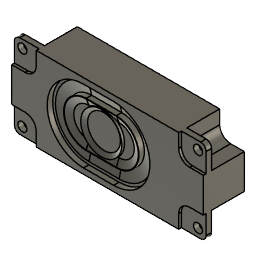
Senso v45 (Autodesk Fusion 360 archive; units mm, degrees)
design "Speaker"
Autodesk Fusion 360 part; units mm, degrees
sketch "Sketch1" plane through (0, 0, 0) normal (0, 1, 0) x (1, 0, 0)
  line L0 (2, 0) -> (68, 0)
  line L1 (70, -2) -> (70, -28.6)
  line L2 (68, -30.6) -> (0, -30.6)
  line L3 (0, -28.6) -> (0, -2)
  circle A0 centre (2.95, -27.65) radius 1.65
  circle A1 centre (2.95, -2.95) radius 1.65
  circle A2 centre (67.05, -27.65) radius 1.65
  circle A3 centre (67.05, -2.95) radius 1.65
  line L4 (2, -30.6) -> (9, -30.6)
  line L5 (9, -30.6) -> (9, -25.6)
  line L6 (5, -21.6) -> (0, -21.6)
  line L7 (0, -21.6) -> (0, -30.6)
  arc A4 (9, -25.6) -> (5, -21.6) centre (5, -25.6) ccw
  line L8 (0, -15.3) -> (70, -15.3) construction
  line L9 (35, -30.6) -> (35, 0) construction
  line L10 (5, -9) -> (0, -9)
  arc A5 (5, -9) -> (9, -5) centre (5, -5) ccw
  line L11 (9, 0) -> (9, -5)
  line L12 (65, -21.6) -> (70, -21.6)
  arc A6 (65, -21.6) -> (61, -25.6) centre (65, -25.6) ccw
  line L13 (61, -30.6) -> (61, -25.6)
  line L14 (65, -9) -> (70, -9)
  arc A7 (61, -5) -> (65, -9) centre (65, -5) ccw
  line L15 (61, 0) -> (61, -5)
  arc A8 (0, -28.6) -> (2, -30.6) centre (2, -28.6) ccw
  arc A9 (2, 0) -> (0, -2) centre (2, -2) ccw
  arc A10 (70, -2) -> (68, 0) centre (68, -2) ccw
  arc A11 (68, -30.6) -> (70, -28.6) centre (68, -28.6) ccw
  line L16 (26.25, -28.55) -> (37.25, -28.55)
  line L17 (37.25, -2.05) -> (26.25, -2.05)
  arc A12 (13, -15.3) -> (26.25, -28.55) centre (26.25, -15.3) ccw
  arc A13 (26.25, -2.05) -> (13, -15.3) centre (26.25, -15.3) ccw
  arc A14 (37.25, -28.55) -> (50.5, -15.3) centre (37.25, -15.3) ccw
  arc A15 (50.5, -15.3) -> (37.25, -2.05) centre (37.25, -15.3) ccw
  arc A16 (18, -15.3) -> (26.25, -23.55) centre (26.25, -15.3) ccw
  line L18 (26.25, -23.55) -> (37.25, -23.55)
  arc A17 (37.25, -23.55) -> (45.5, -15.3) centre (37.25, -15.3) ccw
  arc A18 (45.5, -15.3) -> (37.25, -7.05) centre (37.25, -15.3) ccw
  line L19 (37.25, -7.05) -> (26.25, -7.05)
  arc A19 (26.25, -7.05) -> (18, -15.3) centre (26.25, -15.3) ccw
  arc A20 (14, -15.3) -> (26.25, -27.55) centre (26.25, -15.3) ccw
  line L20 (26.25, -27.55) -> (37.25, -27.55)
  arc A21 (37.25, -27.55) -> (49.5, -15.3) centre (37.25, -15.3) ccw
  arc A22 (49.5, -15.3) -> (37.25, -3.05) centre (37.25, -15.3) ccw
  line L21 (37.25, -3.05) -> (26.25, -3.05)
  arc A23 (26.25, -3.05) -> (14, -15.3) centre (26.25, -15.3) ccw
  line L22 (26.25, -15.3) -> (37.25, -15.3)
  circle A24 centre (31.75, -15.3) radius 7.5
  line L23 (37.25, -7.25) -> (26.25, -7.25)
  arc A25 (26.25, -7.25) -> (18.2, -15.3) centre (26.25, -15.3) ccw
  arc A26 (18.2, -15.3) -> (26.25, -23.35) centre (26.25, -15.3) ccw
  line L24 (26.25, -23.35) -> (37.25, -23.35)
  arc A27 (37.25, -23.35) -> (45.3, -15.3) centre (37.25, -15.3) ccw
  arc A28 (45.3, -15.3) -> (37.25, -7.25) centre (37.25, -15.3) ccw
  circle A29 centre (31.75, -15.3) radius 6
  point P0 (70, 0)
  point P1 (13, -28.55)
  point P2 (50.5, -28.55)
  point P3 (13, -2.05)
  dimension "d1" = 70
  dimension "d2" = 30.6
  dimension "d5" = 3.3
  dimension "d6" = 2.95
  dimension "d7" = 2.95
  dimension "d12" = 3.3
  dimension "d13" = 2.95
  dimension "d14" = 2.95
  dimension "d15" = 3.3
  dimension "d16" = 3.3
  dimension "d17" = 2.95
  dimension "d18" = 2.95
  dimension "d19" = 2.95
  dimension "d20" = 2.95
  dimension "d21" = 9
  dimension "d22" = 9
  dimension "d23" = 4
  dimension "d28" = 2
  dimension "d31" = 37.5
  dimension "d32" = 26.5
  dimension "d34" = 13.25
  dimension "d35" = 13.25
  dimension "d36" = 13.25
  dimension "d37" = 13.25
  dimension "d38" = -5
  dimension "d43" = -1
  dimension "d48" = 15
  dimension "d49" = -0.2
  dimension "d54" = 12
  constraint horizontal L0
  constraint vertical L1
  constraint horizontal L2
  constraint vertical L3
  constraint horizontal L4
  constraint vertical L5
  constraint horizontal L6
  constraint vertical L7
  constraint tangent L6 A4
  constraint tangent L5 A4
  constraint symmetric L4.end L8 L11.start
  constraint symmetric L6.end L8 L10.end
  constraint symmetric L6.start L8 L10.start
  constraint symmetric L5.end L8 A5.end
  constraint symmetric A4 L8 A5
  constraint symmetric L4.end L9 L13.start
  constraint symmetric L6.end L9 L12.end
  constraint symmetric L6.start L9 L12.start
  constraint symmetric L5.end L9 A6.end
  constraint symmetric A4 L9 A6
  constraint symmetric L9 L10.start L14.start
  constraint symmetric L9 L10.end L14.end
  constraint symmetric L9 A5.end A7.start
  constraint symmetric L9 A5 A7
  constraint symmetric L9 L11.start L15.start
  constraint coincident L3 L8.start
  constraint coincident L2.end L4
  constraint tangent L4 A8
  constraint tangent L3 A8
  constraint coincident L0 L9.end
  constraint coincident origin L3
  constraint coincident origin L0
  constraint tangent L3 A9
  constraint tangent L0 A9
  constraint equal A8 A9
  constraint coincident L1 L8.end
  constraint coincident P0 L0
  constraint coincident P0 L1
  constraint tangent L0 A10
  constraint tangent L1 A10
  constraint equal A8 A10
  constraint coincident L2 L9.start
  constraint tangent L1 A11
  constraint tangent L2 A11
  constraint equal A8 A11
  constraint horizontal L16
  constraint horizontal L17
  constraint coincident P1 L16
  constraint tangent L16 A12
  constraint coincident P3 L17
  constraint tangent L17 A13
  constraint coincident A12.start A13.end
  constraint coincident P2 L16
  constraint tangent L16 A14
  constraint tangent L17 A15
  constraint coincident A14.end A15.start
  constraint coincident A12.centre A13.centre
  constraint coincident A14.centre A15.centre
  constraint perpendicular L9 L22
  constraint midpoint L22 A24.centre
  constraint concentric A24 A29
  measures "d1" distance of origin P0
  measures "d2" distance of origin L2.end
  measures "d5" diameter of A0
  measures "d6" distance of L3 A0.centre
  measures "d7" distance of L2 A0.centre
  measures "d12" diameter of A1
  measures "d13" distance of L3 A1.centre
  measures "d14" distance of L0 A1.centre
  measures "d15" diameter of A2
  measures "d16" diameter of A3
  measures "d17" distance of L1 A3.centre
  measures "d18" distance of L0 A3.centre
  measures "d19" distance of L1 A2.centre
  measures "d20" distance of L2 A2.centre
  measures "d21" distance of L2.end L4.end
  measures "d22" distance of L2.end L6.end
  measures "d23" radius of A4
  measures "d28" radius of A8
  measures "d31" distance of P1 P2
  measures "d32" distance of P1 P3
  measures "d34" radius of A12
  measures "d35" radius of A13
  measures "d36" radius of A14
  measures "d37" radius of A15
  measures "d48" diameter of A24
  measures "d54" diameter of A29
extrude "Extrude1" add sketch "Sketch1" along normal blind 15 contours L0 L1 L2 L3 L5 L6 A4 L10 A5 L11 L12 A6 L13 L14 A7 L15 | L16 L17 A12 A13 A14 A15 | A16 L18 A17 A18 L19 A19 | A20 L20 A21 A22 L21 A23 | A24 | L23 A25 A26 L24 A27 A28 | A29
extrude "Extrude2" add sketch "Sketch1" along normal blind 3 contours L0 L3 L10 A5 L11 A9 | L0 L1 L14 A7 L15 A10 | L2 L3 L4 L5 L6 L7 A4 A8 | L1 L2 L12 A6 L13 A11
extrude "Extrude3" cut sketch "Sketch1" along normal blind 1 contours L0 L3 L10 A5 L11 A9 | L0 L1 L14 A7 L15 A10 | L2 L3 L4 L5 L6 L7 A4 A8 | L1 L2 L12 A6 L13 A11
extrude "Extrude4" cut sketch "Sketch1" along normal blind 2 contours L16 L17 A12 A13 A14 A15 | A20 L20 A21 A22 L21 A23
extrude "Extrude5" cut sketch "Sketch1" along normal blind 1 contours A16 L18 A17 A18 L19 A19 | A24 | L23 A25 A26 L24 A27 A28 | A29
extrude "Extrude6" cut sketch "Sketch1" along normal blind 3 contours A20 L20 A21 A22 L21 A23
chamfer "Chamfer1" distance 1 distance2 4 4 edges at (31.75, 3, 27.55) (49.5, 3, 15.3) (31.75, 3, 3.05) (14, 3, 15.3) measured on face at (29.9167, 2.3333, 27.55) measured on face at (45.1241, 2.6667, 24.684) measured on face at (33.5833, 2.3333, 3.05) measured on face at (17.0652, 2.3333, 23.4057)
extrude "Extrude7" cut sketch "Sketch1" along normal blind 2 contours L23 A25 A26 L24 A27 A28
chamfer "Chamfer2" distance 1 distance2 2.5 4 edges at (31.75, 2, 23.35) (45.3, 2, 15.3) (31.75, 2, 7.25) (18.2, 2, 15.3) measured on face at (29.9167, 1.3333, 23.35) measured on face at (38.0515, 1.3333, 7.29) measured on face at (33.5833, 1.3333, 7.25) measured on face at (18.5009, 1.3333, 17.4803)
extrude "Extrude8" cut sketch "Sketch1" along normal blind 2 contours A29
chamfer "Chamfer3" distance 1.5 distance2 1 1 edges at (26.156, 1, 17.4697) measured on face at (38.7221, 1, 14.9274)
equation "d6 = 1.3 mm + ( 3.3 / 2 ) * 1 mm"
equation "d34 = ( 26.5 / 2 ) * 1 mm"
equation "d35 = ( 26.5 / 2 ) * 1 mm"
equation "d36 = ( 26.5 / 2 ) * 1 mm"
equation "d37 = ( 26.5 / 2 ) * 1 mm"
equation "d54 = 15 mm - 3 mm"

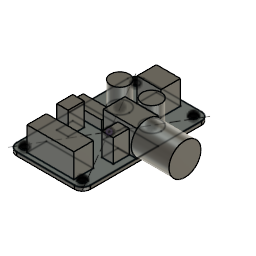
design "Fasizi AudioVerstaerker PAM8406"
Autodesk Fusion 360 part; units mm, degrees
sketch "Sketch1" plane through (0, 0, 0) normal (0, 0, 1) x (1, 0, 0)
  line L0 (12.63, 27.8) -> (-12.63, 27.8)
  line L1 (-16.13, 24.3) -> (-16.13, -24.3)
  line L2 (-12.63, -27.8) -> (12.63, -27.8)
  line L3 (16.13, -24.3) -> (16.13, 24.3)
  line L4 (16.13, 27.8) -> (-16.13, -27.8) construction
  line L5 (-16.13, 27.8) -> (16.13, -27.8) construction
  circle A0 centre (-12.63, 24.3) radius 1.5
  circle A1 centre (12.63, 24.3) radius 1.5
  circle A2 centre (-12.63, -24.3) radius 1.5
  circle A3 centre (12.63, -24.3) radius 1.5
  arc A4 (-12.63, 27.8) -> (-16.13, 24.3) centre (-12.63, 24.3) ccw
  arc A5 (16.13, 24.3) -> (12.63, 27.8) centre (12.63, 24.3) ccw
  arc A6 (12.63, -27.8) -> (16.13, -24.3) centre (12.63, -24.3) ccw
  arc A7 (-16.13, -24.3) -> (-12.63, -27.8) centre (-12.63, -24.3) ccw
  line L6 (-4.63, 25.3) -> (5.87, 25.3)
  line L7 (5.87, 25.3) -> (5.87, 16.8)
  line L8 (5.87, 16.8) -> (-4.63, 16.8)
  line L9 (-4.63, 16.8) -> (-4.63, 25.3)
  circle A8 centre (-6.98, 11.65) radius 4.15
  circle A9 centre (6.98, 11.65) radius 4.15
  line L10 (-16.13, 4.8) -> (-2.13, 4.8)
  line L11 (-2.13, 4.8) -> (-2.13, -1.2)
  line L12 (-2.13, -1.2) -> (-16.13, -1.2)
  line L13 (-16.13, -1.2) -> (-16.13, 4.8)
  line L14 (16.13, 5.3) -> (1.63, 5.3)
  line L15 (1.63, 5.3) -> (1.63, -4.2)
  line L16 (1.63, -4.2) -> (16.13, -4.2)
  line L17 (16.13, -4.2) -> (16.13, 5.3)
  line L18 (-12.13, -3.8) -> (-7.13, -3.8)
  line L19 (-7.13, -3.8) -> (-7.13, -10.8)
  line L20 (-7.13, -10.8) -> (-12.13, -10.8)
  line L21 (-12.13, -10.8) -> (-12.13, -3.8)
  line L22 (8.13, -11.3) -> (13.13, -11.3)
  line L23 (13.13, -11.3) -> (13.13, -4.3)
  line L24 (13.13, -4.3) -> (8.13, -4.3)
  line L25 (8.13, -4.3) -> (8.13, -11.3)
  line L26 (-10.13, -17.3) -> (10.37, -17.3)
  line L27 (10.37, -17.3) -> (10.37, -25.8)
  line L28 (10.37, -25.8) -> (-10.13, -25.8)
  line L29 (-10.13, -25.8) -> (-10.13, -17.3)
  dimension "d1" = 32.26
  dimension "d2" = 55.6
  dimension "d3" = 3
  dimension "d4" = 3.5
  dimension "d5" = 3.5
  dimension "d8" = 25.26
  dimension "d9" = -48.6
  dimension "d10" = 3.5
  dimension "d13" = 10.5
  dimension "d14" = 8.5
  dimension "d15" = 11.5
  dimension "d16" = 2.5
  dimension "d19" = 8.3
  dimension "d20" = 8.3
  dimension "d21" = 9.15
  dimension "d22" = 9.15
  dimension "d23" = 16.15
  dimension "d24" = 16.15
  dimension "d27" = 14
  dimension "d28" = 6
  dimension "d29" = 23
  dimension "d32" = 14.5
  dimension "d33" = 9.5
  dimension "d36" = 5
  dimension "d37" = 7
  dimension "d38" = 4
  dimension "d39" = 17
  dimension "d40" = 22.5
  dimension "d41" = 5
  dimension "d42" = 7
  dimension "d43" = 3
  dimension "d44" = 16.5
  dimension "d47" = 20.5
  dimension "d48" = 8.5
  dimension "d49" = 6
  dimension "d52" = 2
  constraint horizontal L0
  constraint perpendicular L0 L1
  constraint parallel L0 L2
  constraint parallel L1 L3
  constraint coincident L4 origin
  constraint coincident L5 origin
  constraint coincident L5.start L1
  constraint coincident L5.start L0
  constraint tangent L1 A4
  constraint tangent L0 A4
  constraint coincident L4.start L0
  constraint coincident L4.start L3
  constraint tangent L0 A5
  constraint tangent L3 A5
  constraint equal A4 A5
  constraint coincident L5.end L3
  constraint coincident L5.end L2
  constraint tangent L3 A6
  constraint tangent L2 A6
  constraint equal A4 A6
  constraint coincident L4.end L1
  constraint coincident L4.end L2
  constraint tangent L1 A7
  constraint tangent L2 A7
  constraint equal A4 A7
  constraint horizontal L6
  constraint vertical L7
  constraint horizontal L8
  constraint vertical L9
  constraint horizontal L10
  constraint vertical L11
  constraint horizontal L12
  constraint vertical L13
  constraint coincident L1 L10.start
  constraint horizontal L14
  constraint vertical L15
  constraint horizontal L16
  constraint vertical L17
  constraint coincident L3 L14.start
  constraint horizontal L18
  constraint vertical L19
  constraint horizontal L20
  constraint vertical L21
  constraint horizontal L22
  constraint vertical L23
  constraint horizontal L24
  constraint vertical L25
  constraint horizontal L26
  constraint vertical L27
  constraint horizontal L28
  constraint vertical L29
  measures "d1" distance of L4.end L5.end
  measures "d2" distance of L5.start L4.end
  measures "d3" diameter of A0
  measures "d4" distance of L1 A0.centre
  measures "d5" distance of L0 A0.centre
  measures "d10" radius of A4
  measures "d13" distance of L6.start L6.end
  measures "d14" distance of L6.start L8.end
  measures "d15" distance of L1 L9
  measures "d16" distance of L0 L6
  measures "d19" diameter of A8
  measures "d20" diameter of A9
  measures "d21" distance of L1 A8.centre
  measures "d22" distance of L3 A9.centre
  measures "d23" distance of L0 A9.centre
  measures "d24" distance of L0 A8.centre
  measures "d27" distance of L10.start L10.end
  measures "d28" distance of L10.start L12.end
  measures "d29" distance of L0 L10
  measures "d32" distance of L14.start L14.end
  measures "d33" distance of L14.start L16.end
  measures "d36" distance of L18.start L18.end
  measures "d37" distance of L18.start L20.end
  measures "d38" distance of L1 L21
  measures "d39" distance of L2 L20
  measures "d40" distance of L0 L14
  measures "d41" distance of L22.start L22.end
  measures "d42" distance of L22.start L24.end
  measures "d43" distance of L3 L23
  measures "d44" distance of L2 L22
  measures "d47" distance of L26.start L26.end
  measures "d48" distance of L26.start L28.end
  measures "d49" distance of L1 L29
  measures "d52" distance of L2 L28
extrude "Extrude1" add sketch "Sketch1" against normal blind 1.6 contours L0 L1 L2 L3 A4 A5 A6 A7 L10 L11 L12 L14 L15 L16 | L3 L14 L15 L16 L17 | L1 L10 L11 L12 L13 | L6 L7 L8 L9 | A8 | A9 | L18 L19 L20 L21 | L22 L23 L24 L25 | L26 L27 L28 L29 makes body 1
extrude "Extrude2" add sketch "Sketch1" along normal blind 10.5 separate body contours L6 L7 L8 L9 makes body 2
extrude "Extrude3" add sketch "Sketch1" along normal blind 10.5 separate body contours A8 | A9 makes body 3 at (-2.8352, 11.4431, 7) makes body 4 at (11.1248, 11.4431, 7)
extrude "Extrude4" add sketch "Sketch1" along normal blind 4 separate body contours L1 L10 L11 L12 L13 makes body 5
extrude "Extrude5" add sketch "Sketch1" along normal blind 11.5 separate body contours L3 L14 L15 L16 L17 makes body 6
extrude "Extrude6" add sketch "Sketch1" along normal blind 10 separate body contours L18 L19 L20 L21 | L22 L23 L24 L25 makes body 7 at (13.13, -8.9667, 3.3333) makes body 8 at (-7.13, -6.1333, 3.3333)
extrude "Extrude7" add sketch "Sketch1" along normal blind 10.5 separate body contours L26 L27 L28 L29 makes body 9
sketch "Sketch2" plane through (16.13, 0, 0) normal (1, 0, 0) x (0, 1, 0)
  line L0 (-4.2, 0) -> (5.3, 0)
  line L1 (5.3, 0) -> (5.3, 11.5)
  line L2 (5.3, 11.5) -> (-4.2, 11.5)
  line L3 (-4.2, 11.5) -> (-4.2, 0)
  circle A0 centre (0.55, 5.75) radius 7
  dimension "d55" = 14
  measures "d55" diameter of A0
extrude "Extrude8" add sketch "Sketch2" along normal blind 16.5 contours L0 L1 L2 L3 A0 | L0 A0 | L3 A0 | L1 A0 | L2 A0 bodies 1 6
equation "d4 = 2 mm + 1.5 mm"
equation "d5 = 2 mm + 1.5 mm"
equation "d8 = 32.26 mm - ( 3.5 * 2 ) * 1 mm"
equation "d9 = -55.6 mm + ( 3.5 * 2 ) * 1 mm"
equation "d21 = 5 mm + ( 8.3 / 2 ) * 1 mm"
equation "d23 = 12 mm + ( 8.3 / 2 ) * 1 mm"

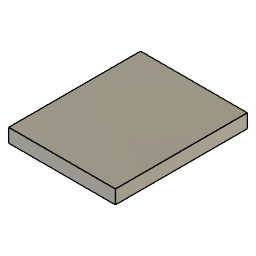
design "LP605060JU Akku"
Autodesk Fusion 360 part; units mm, degrees
sketch "Sketch1" plane through (0, 0, 0) normal (0, 0, 1) x (1, 0, 0)
  line L0 (0, 0) -> (51, 0)
  line L1 (51, 0) -> (51, 63)
  line L2 (51, 63) -> (0, 63)
  line L3 (0, 63) -> (0, 0)
  dimension "d1" = 51
  dimension "d2" = 63
  constraint horizontal L0
  constraint vertical L1
  constraint horizontal L2
  constraint vertical L3
  constraint coincident L0.start L3.end
  measures "d1" distance of L0.start L0.end
  measures "d2" distance of L0.start L2.end
extrude "Extrude1" add sketch "Sketch1" along normal blind 6.6

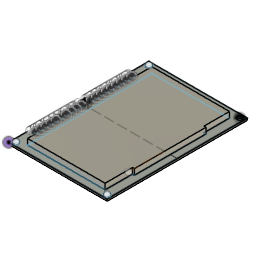
design "COM-OLED 2.42"
Autodesk Fusion 360 part; units mm, degrees
sketch "Sketch1" plane through (0, 0, 0) normal (0, 0, 1) x (1, 0, 0)
  line L0 (0, 0) -> (49.5, 0)
  line L1 (49.5, 0) -> (49.5, 70.5)
  line L2 (49.5, 70.5) -> (0, 70.5)
  line L3 (0, 70.5) -> (0, 0)
  circle A0 centre (47.65, 68.65) radius 1.3
  circle A1 centre (47.65, 1.85) radius 1.3
  circle A2 centre (1.85, 68.65) radius 1.3
  circle A3 centre (1.85, 1.85) radius 1.3
  line L4 (45, 66) -> (6, 66)
  line L5 (6, 66) -> (6, 3.5)
  line L6 (6, 3.5) -> (45, 3.5)
  line L7 (46, 17.25) -> (46, 53.25)
  line L8 (0, 35.25) -> (49.5, 35.25) construction
  line L9 (0, 37.32) -> (2.6, 37.32)
  line L10 (2.6, 37.32) -> (2.6, 35.72)
  line L11 (2.6, 35.72) -> (0, 35.72)
  circle A4 centre (2.6, 36.52) radius 0.8
  circle A5 centre (2.6, 33.98) radius 0.8
  line L12 (2.6, 34.78) -> (2.6, 33.18)
  line L13 (2.6, 33.18) -> (0, 33.18)
  line L14 (0, 34.78) -> (2.6, 34.78)
  line L15 (2.6, 36.52) -> (0, 36.52) construction
  line L16 (2.6, 33.98) -> (0, 33.98) construction
  line L17 (2.6, 38.26) -> (0, 38.26)
  circle A6 centre (2.6, 39.06) radius 0.8
  line L18 (2.6, 39.06) -> (0, 39.06) construction
  line L19 (0, 39.86) -> (2.6, 39.86)
  circle A7 centre (2.6, 41.6) radius 0.8
  line L20 (2.6, 41.6) -> (0, 41.6) construction
  line L21 (2.6, 40.8) -> (0, 40.8)
  line L22 (0, 42.4) -> (2.6, 42.4)
  line L23 (0, 44.94) -> (2.6, 44.94)
  circle A8 centre (2.6, 44.14) radius 0.8
  line L24 (2.6, 44.14) -> (0, 44.14) construction
  line L25 (2.6, 43.34) -> (0, 43.34)
  line L26 (2.6, 46.68) -> (0, 46.68) construction
  line L27 (0, 47.48) -> (2.6, 47.48)
  circle A9 centre (2.6, 46.68) radius 0.8
  line L28 (2.6, 45.88) -> (0, 45.88)
  line L29 (2.6, 49.22) -> (0, 49.22) construction
  line L30 (2.6, 48.42) -> (0, 48.42)
  line L31 (0, 50.02) -> (2.6, 50.02)
  line L32 (2.6, 53.5) -> (0, 53.5)
  line L33 (0, 57.64) -> (2.6, 57.64)
  line L34 (0, 55.1) -> (2.6, 55.1)
  circle A10 centre (2.6, 54.3) radius 0.8
  line L35 (2.6, 56.04) -> (0, 56.04)
  circle A11 centre (2.6, 49.22) radius 0.8
  line L36 (0, 52.56) -> (2.6, 52.56)
  line L37 (2.6, 51.76) -> (0, 51.76) construction
  line L38 (2.6, 50.96) -> (0, 50.96)
  circle A12 centre (2.6, 51.76) radius 0.8
  line L39 (2.6, 54.3) -> (0, 54.3) construction
  circle A13 centre (2.6, 56.84) radius 0.8
  line L40 (2.6, 56.84) -> (0, 56.84) construction
  line L41 (2.6, 59.38) -> (0, 59.38) construction
  line L42 (0, 60.18) -> (2.6, 60.18)
  circle A14 centre (2.6, 59.38) radius 0.8
  line L43 (2.6, 58.58) -> (0, 58.58)
  line L44 (2.6, 10.32) -> (0, 10.32)
  circle A15 centre (2.6, 11.12) radius 0.8
  circle A16 centre (2.6, 21.28) radius 0.8
  line L45 (2.6, 13.66) -> (0, 13.66) construction
  line L46 (2.6, 25.56) -> (0, 25.56)
  circle A17 centre (2.6, 28.9) radius 0.8
  line L47 (0, 11.92) -> (2.6, 11.92)
  line L48 (2.6, 20.48) -> (0, 20.48)
  circle A18 centre (2.6, 18.74) radius 0.8
  line L49 (0, 14.46) -> (2.6, 14.46)
  line L50 (0, 19.54) -> (2.6, 19.54)
  line L51 (0, 17) -> (2.6, 17)
  line L52 (2.6, 15.4) -> (0, 15.4)
  line L53 (2.6, 11.12) -> (0, 11.12) construction
  circle A19 centre (2.6, 13.66) radius 0.8
  circle A20 centre (2.6, 23.82) radius 0.8
  line L54 (2.6, 28.1) -> (0, 28.1)
  line L55 (0, 24.62) -> (2.6, 24.62)
  circle A21 centre (2.6, 26.36) radius 0.8
  line L56 (0, 32.24) -> (2.6, 32.24)
  line L57 (2.6, 23.02) -> (0, 23.02)
  line L58 (2.6, 31.44) -> (0, 31.44) construction
  circle A22 centre (2.6, 31.44) radius 0.8
  line L59 (0, 22.08) -> (2.6, 22.08)
  line L60 (2.6, 17.94) -> (0, 17.94)
  circle A23 centre (2.6, 16.2) radius 0.8
  line L61 (2.6, 16.2) -> (0, 16.2) construction
  line L62 (2.6, 21.28) -> (0, 21.28) construction
  line L63 (2.6, 23.82) -> (0, 23.82) construction
  line L64 (0, 27.16) -> (2.6, 27.16)
  line L65 (2.6, 26.36) -> (0, 26.36) construction
  line L66 (0, 29.7) -> (2.6, 29.7)
  line L67 (2.6, 28.9) -> (0, 28.9) construction
  line L68 (2.6, 12.86) -> (0, 12.86)
  line L69 (2.6, 18.74) -> (0, 18.74) construction
  line L70 (2.6, 30.64) -> (0, 30.64)
  line L71 (46, 53.25) -> (45, 53.25)
  line L72 (45, 53.25) -> (45, 66)
  line L73 (43.0482, 35.25) -> (43.0482, 17.25) construction
  line L74 (46, 17.25) -> (45, 17.25)
  line L75 (45, 17.25) -> (45, 3.5)
  dimension "d1" = 49.5
  dimension "d2" = 70.5
  dimension "d3" = 2.6
  dimension "d4" = 2.6
  dimension "d5" = 66.8
  dimension "d6" = 2.6
  dimension "d7" = 2.6
  dimension "d8" = 66.8
  dimension "d9" = 45.8
  dimension "d10" = 1.85
  dimension "d11" = 1.85
  dimension "d14" = 3.5
  dimension "d15" = 2.6
  dimension "d16" = 1.6
  dimension "d17" = 2.6
  dimension "d18" = 1.6
  dimension "d19" = 2.54
  dimension "d20" = 1.27
  dimension "d21" = 2.6
  dimension "d22" = 1.6
  dimension "d23" = 2.6
  dimension "d24" = 1.6
  dimension "d25" = 2.6
  dimension "d26" = 1.6
  dimension "d27" = 2.6
  dimension "d28" = 1.6
  dimension "d29" = 2.6
  dimension "d30" = 1.6
  dimension "d31" = 2.6
  dimension "d32" = 1.6
  dimension "d33" = 2.6
  dimension "d34" = 1.6
  dimension "d35" = 2.6
  dimension "d36" = 1.6
  dimension "d37" = 2.6
  dimension "d38" = 1.6
  dimension "d39" = 2.6
  dimension "d40" = 1.6
  dimension "d41" = 2.6
  dimension "d42" = 1.6
  dimension "d43" = 2.6
  dimension "d44" = 1.6
  dimension "d45" = 2.6
  dimension "d46" = 1.6
  dimension "d47" = 2.6
  dimension "d48" = 1.6
  dimension "d49" = 2.6
  dimension "d50" = 1.6
  dimension "d51" = 2.6
  dimension "d52" = 1.6
  dimension "d53" = 2.6
  dimension "d54" = 1.6
  dimension "d55" = 2.6
  dimension "d56" = 1.6
  dimension "d58" = 1
  dimension "d59" = 18
  dimension "d60" = 1
  constraint horizontal L0
  constraint vertical L1
  constraint horizontal L2
  constraint vertical L3
  constraint coincident L0.start L3.end
  constraint horizontal L4
  constraint vertical L5
  constraint horizontal L6
  constraint vertical L7
  constraint midpoint L3 L8.start
  constraint midpoint L1 L8.end
  constraint coincident L3 L9.start
  constraint perpendicular L3 L9
  constraint perpendicular L9 L10
  constraint coincident L3 L11.end
  constraint perpendicular L3 L11
  constraint midpoint L10 A4.centre
  constraint coincident L10.end A4
  constraint perpendicular L12 L14
  constraint midpoint A5.centre L12
  constraint coincident L12.end A5
  constraint coincident A4.centre L15.start
  constraint coincident L3 L15.end
  constraint perpendicular L3 L15
  constraint coincident A5.centre L16.start
  constraint coincident L3 L16.end
  constraint perpendicular L3 L16
  constraint coincident L17.start A6
  constraint coincident A6.centre L18.start
  constraint coincident L21.start A7
  constraint coincident A7.centre L20.start
  constraint coincident L25.start A8
  constraint coincident A8.centre L24.start
  constraint coincident L28.start A9
  constraint coincident L26.start A9.centre
  constraint coincident L30.start A11
  constraint coincident L29.start A11.centre
  constraint coincident L38.start A12
  constraint coincident L37.start A12.centre
  constraint coincident L32.start A10
  constraint coincident A10.centre L39.start
  constraint coincident L35.start A13
  constraint coincident A13.centre L40.start
  constraint coincident L43.start A14
  constraint coincident L41.start A14.centre
  constraint coincident L44.start A15
  constraint coincident A15.centre L53.start
  constraint coincident L68.start A19
  constraint coincident L45.start A19.centre
  constraint coincident L52.start A23
  constraint coincident A23.centre L61.start
  constraint coincident L60.start A18
  constraint coincident A18.centre L69.start
  constraint coincident L48.start A16
  constraint coincident A16.centre L62.start
  constraint coincident L57.start A20
  constraint coincident A20.centre L63.start
  constraint coincident L46.start A21
  constraint coincident A21.centre L65.start
  constraint coincident L54.start A17
  constraint coincident A17.centre L67.start
  constraint coincident L70.start A22
  constraint coincident L58.start A22.centre
  constraint coincident L8 L73.start
  constraint perpendicular L7 L71
  constraint perpendicular L4 L72
  constraint perpendicular L8 L73
  constraint perpendicular L7 L74
  constraint perpendicular L6 L75
  measures "d1" distance of L0.start L0.end
  measures "d2" distance of L0.start L2.end
  measures "d3" diameter of A0
  measures "d4" diameter of A1
  measures "d5" distance of A0.centre A1.centre
  measures "d6" diameter of A2
  measures "d7" diameter of A3
  measures "d8" distance of A2.centre A3.centre
  measures "d9" distance of A0.centre A2.centre
  measures "d10" distance of L2 A0.centre
  measures "d11" distance of L1 A0.centre
  measures "d14" distance of L1 L7
  measures "d15" distance of L9.start L9.end
  measures "d16" distance of L9.end L10.end
  measures "d17" distance of L12.start L14.start
  measures "d18" distance of L12.end L12.start
  measures "d19" distance of L15 L16
  measures "d20" distance of L8 L15
  measures "d21" distance of L19.end L19.start
  measures "d22" distance of L17.start L19.end
  measures "d23" distance of L22.end L22.start
  measures "d24" distance of L22.end L21.start
  measures "d25" distance of L23.end L23.start
  measures "d26" distance of L23.end L25.start
  measures "d27" distance of L27.end L27.start
  measures "d28" distance of L27.end L28.start
  measures "d29" distance of L31.end L31.start
  measures "d30" distance of L31.end L30.start
  measures "d31" distance of L36.end L36.start
  measures "d32" distance of L36.end L38.start
  measures "d33" distance of L34.end L34.start
  measures "d34" distance of L34.end L32.start
  measures "d35" distance of L33.end L33.start
  measures "d36" distance of L33.end L35.start
  measures "d37" distance of L42.start L42.end
  measures "d38" distance of L42.end L43.start
  measures "d39" distance of L47.end L47.start
  measures "d40" distance of L47.end L44.start
  measures "d41" distance of L49.end L49.start
  measures "d42" distance of L49.end L68.start
  measures "d43" distance of L51.end L51.start
  measures "d44" distance of L51.end L52.start
  measures "d45" distance of L50.end L50.start
  measures "d46" distance of L50.end L60.start
  measures "d47" distance of L59.end L59.start
  measures "d48" distance of L59.end L48.start
  measures "d49" distance of L55.start L55.end
  measures "d50" distance of L57.start L55.end
  measures "d51" distance of L64.start L64.end
  measures "d52" distance of L64.end L46.start
  measures "d53" distance of L66.start L66.end
  measures "d54" distance of L66.end L54.start
  measures "d55" distance of L56.start L56.end
  measures "d56" distance of L70.start L56.end
  measures "d58" distance of L7.end L71.end
  measures "d59" distance of L73.start L73.end
  measures "d60" distance of L7.start L74.end
extrude "Extrude1" add sketch "Sketch1" against normal blind 1 contours L0 L1 L2 L3 L9 L11 A4 A5 L13 L14 L17 A6 L19 A7 L21 L22 L23 A8 L25 L27 A9 L28 L30 L31 L32 L33 L34 A10 L35 A11 L36 L38 A12 A13 L42 A14 L43 L44 A15 A16 L46 A17 L47 L48 A18 L49 L50 L51 L52 A19 A20 L54 L55 A21 L56 L57 A22 L59 L60 A23 L64 L66 L68 L70 | L3 L44 A15 L47 | L3 L49 A19 L68 | L3 L42 A14 L43 | L3 L51 L52 A23 | L3 L33 L35 A13 | L3 A18 L50 L60 | L3 L32 L34 A10 | L3 A16 L48 L59 | L3 L36 L38 A12 | L3 A20 L55 L57 | L3 L30 L31 A11 | L3 L46 A21 L64 | L3 L27 A9 L28 | L3 A17 L54 L66 | L3 L23 A8 L25 | L3 L56 A22 L70 | L3 A7 L21 L22 | L3 A5 L13 L14 | L3 L17 A6 L19 | L3 L9 L11 A4 | L4 L5 L6 L7 L71 L72 L74 L75
extrude "Extrude2" add sketch "Sketch1" along normal blind 2.9 contours L4 L5 L6 L7 L71 L72 L74 L75
extrude "Extrude3" cut sketch "Sketch1" against normal blind 0.1 contours L3 L44 A15 L47 | L3 L49 A19 L68 | L3 L42 A14 L43 | L3 L51 L52 A23 | L3 L33 L35 A13 | L3 A18 L50 L60 | L3 L32 L34 A10 | L3 A16 L48 L59 | L3 L36 L38 A12 | L3 A20 L55 L57 | L3 L30 L31 A11 | L3 L46 A21 L64 | L3 L27 A9 L28 | L3 A17 L54 L66 | L3 L23 A8 L25 | L3 L56 A22 L70 | L3 A7 L21 L22 | L3 A5 L13 L14 | L3 L17 A6 L19 | L3 L9 L11 A4
